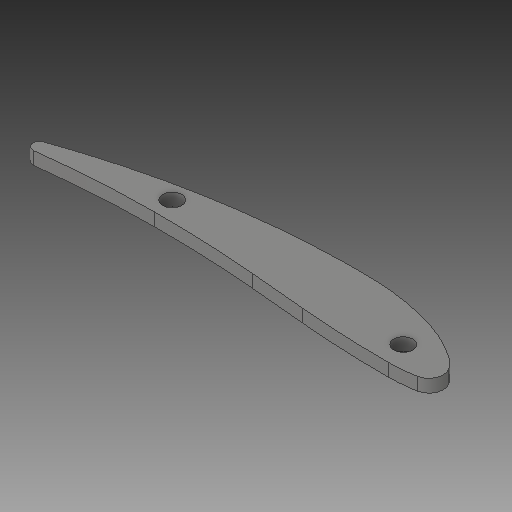
# Autodesk Inventor part: plate_sf2
Saved by Autodesk Inventor 2018.2 (Build 222227000, 227)
## iProperties
Created: 2018-03-05
Part Number: plate_sf2
Material: 木材 (オーク)
Document SubType Name: Modeling
Designer: ku_sk
Density: 0.76 g/cm^3
Appearance: ホワイト オーク材 - ナチュラル 標準の光沢
Author: ku_sk
Autodesk Inventor part; units mm, degrees
ref_plane "YZ Plane" through (0, 0, 0) normal (1, 0, 0) x (0, 1, 0)
ref_plane "XZ Plane" through (0, 0, 0) normal (0, 1, 0) x (-1, 0, 0)
ref_plane "XY Plane" through (0, 0, 0) normal (0, 0, 1) x (1, 0, 0)
sketch "スケッチ1" plane through (0, 0, 0) normal (0, 1, 0) x (-1, 0, 0)
  arc A0 (120.7701, -0.6068) -> (119.8564, 3.2634) centre (120.103, 1.2786) ccw projected
  arc A1 (41.4452, -14.9694) -> (120.7701, -0.6068) centre (36.8758, 236.5065) ccw projected
  arc A2 (30.7183, -14.8468) -> (41.4452, -14.9694) centre (38.1525, 166.2425) ccw projected
  arc A3 (11.0166, -11.3447) -> (30.7183, -14.8468) centre (33.77, 59.49) ccw projected
  arc A4 (-0.3565, -5.7585) -> (11.0166, -11.3447) centre (24.3575, 30.1875) ccw projected
  arc A5 (-3.5852, -2.6234) -> (-0.3565, -5.7585) centre (7.25, 5.305) ccw projected
  arc A6 (-0.7848, 4.3726) -> (-3.5852, -2.6234) centre (0, 0) ccw projected
  arc A7 (7.6183, 5.1344) -> (-0.7848, 4.3726) centre (7.775, -43.32) ccw projected
  arc A8 (35.5607, 3.8888) -> (7.6183, 5.1344) centre (8.565, -287.665) ccw projected
  arc A9 (35.5607, 3.8888) -> (52.6853, 2.3311) centre (526.9475, 5310.875) ccw projected
  arc A10 (52.6853, 2.3311) -> (84.6244, 0.9905) centre (82.86, 340.0849) ccw projected
  arc A11 (84.6244, 0.9905) -> (119.8564, 3.2634) centre (83.0725, 299.245) ccw projected
extrude "押し出し1" add sketch "スケッチ1" along normal blind 4
sketch "スケッチ2" plane through (0, 0, 0) normal (0, -1, 0) x (1, 0, 0)
  circle A0 centre (-10, -2) radius 3
  circle A1 centre (-85, -5) radius 3
  point P0 (0, 0)
  dimension "d3" = 6
  dimension "d4" = 6
  dimension "d5" = 10
  dimension "d6" = 2
  dimension "d7" = 5
  dimension "d8" = 85
  constraints: 2 centre point
  measures "d3" diameter of A1
  measures "d4" diameter of A0
  measures "d5" horizontal distance of point (0, 0) A0.centre
  measures "d6" vertical distance of point (0, 0) A0.centre
  measures "d7" vertical distance of point (0, 0) A1.centre
  measures "d8" horizontal distance of point (0, 0) A1.centre
extrude "押し出し2" cut sketch "スケッチ2" against normal through all
equation "\"d4\" = d3"
